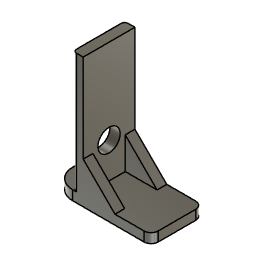
Improved Part (Autodesk Fusion 360 design; units mm, degrees)
Autodesk Fusion 360 part; units mm, degrees
sketch "Skizze1" plane through (0, 0, 0) normal (0, 0, 1) x (1, 0, 0)
  line L0 (-75, 50) -> (-47.27, 50)
  line L1 (-47.27, 50) -> (-47.27, 35.3603)
  line L2 (-47.27, 35.3603) -> (-75, 35.3603)
  line L3 (-75, 35.3603) -> (-75, 50)
  line L4 (-69.4, 50) -> (-69.4, 35.3603)
  line L5 (-66.5, 50) -> (-66.5, 35.3603)
  dimension "d1" = 27.73
  dimension "d2" = 5.6
  dimension "d3" = 2.9
  constraint horizontal L0
  constraint vertical L1
  constraint horizontal L2
  constraint vertical L3
  constraint coincident L0 L4.start
  constraint coincident L2 L4.end
  constraint perpendicular L2 L4
  constraint coincident L0 L5.start
  constraint coincident L2 L5.end
  constraint perpendicular L2 L5
  measures "d1" distance of L0.start L0.end
  measures "d2" distance of L3 L4
  measures "d3" distance of L4 L5
extrude "Extrusion1" add sketch "Skizze1" along normal blind 2.7 contours L0 L2 L3 L4 | L0 L1 L2 L5 makes body 1 at (-73.1333, 45.1201, 0) makes body 2 at (-60.09, 45.1201, 0)
extrude "Extrusion2" add sketch "Skizze1" along normal blind 36.7 contours L0 L2 L4 L5 bodies 1 2
sketch "Skizze2" plane through (-69.4, 0, 0) normal (-1, 0, 0) x (0, -1, 0)
  line L0 (-50, 2.7) -> (-35.3603, 2.7)
  line L1 (-35.3603, 2.7) -> (-35.3603, 36.7)
  line L2 (-35.3603, 36.7) -> (-50, 36.7)
  line L3 (-50, 36.7) -> (-50, 2.7)
  line L4 (-42.6802, 2.7) -> (-42.6802, 36.7) construction
  line L5 (-50, 12.7) -> (-35.3603, 12.7) construction
  line L6 (-50, 2.7) -> (-35.3603, 2.7) construction
  circle A0 centre (-42.6802, 12.7) radius 3.15
  dimension "d8" = 10
  dimension "d9" = 6.3
  constraint midpoint L0 L4.start
  constraint midpoint L2 L4.end
  constraint coincident L3 L5.start
  constraint coincident L1 L5.end
  constraint perpendicular L1 L5
  constraint midpoint L5 A0.centre
  measures "d8" distance of L5 L6
  measures "d9" diameter of A0
extrude "Extrusion3" cut sketch "Skizze2" against normal blind 3 contours A0 bodies 1
fillet "Abrundung1" radius 5.5 2 edges at (-75, 50, 1.35) (-75, 35.3603, 1.35) on bodies 1
sketch "Skizze3" plane through (0, 0, 2.7) normal (0, 0, 1) x (-1, 0, 0)
  line L0 (47.27, -50) -> (66.5, -50)
  line L1 (66.5, -50) -> (66.5, -35.3603)
  line L2 (66.5, -35.3603) -> (47.27, -35.3603)
  line L3 (47.27, -35.3603) -> (47.27, -50)
  line L4 (66.5, -38.1003) -> (47.27, -38.1003)
  line L5 (47.27, -47.26) -> (66.5, -47.26)
  line L6 (57.5, -38.1003) -> (57.5, -35.3603)
  line L7 (57.5, -47.26) -> (57.5, -50)
  dimension "d14" = 2.74
  dimension "d15" = 2.74
  dimension "d16" = 9
  dimension "d17" = 9
  constraint coincident L1 L4.start
  constraint coincident L3 L4.end
  constraint perpendicular L3 L4
  constraint coincident L3 L5.start
  constraint coincident L1 L5.end
  constraint perpendicular L1 L5
  constraint coincident L4 L6.start
  constraint coincident L2 L6.end
  constraint perpendicular L2 L6
  constraint coincident L5 L7.start
  constraint coincident L0 L7.end
  constraint perpendicular L0 L7
  measures "d14" distance of L2 L4
  measures "d15" distance of L0 L5
  measures "d16" distance of L1 L7
  measures "d17" distance of L1 L6
extrude "Extrusion4" add sketch "Skizze3" along normal blind 9 contours L0 L1 L5 L7 | L1 L2 L4 L6 bodies 1
chamfer "Fase2" distance 9 angle 45 2 edges at (-57.5, 36.7303, 11.7) (-57.5, 48.63, 11.7) on bodies 1
fillet "Abrundung2" radius 1 2 edges at (-69.4, 50, 19.7) (-69.4, 35.3603, 19.7) on bodies 1
fillet "Abrundung3" radius 2 2 edges at (-47.27, 50, 1.35) (-47.27, 35.3603, 1.35) on bodies 1
equation "d1 = 20 mm + 7.73 mm"
equation "d6 = 34 mm + 2.7 mm"
equation "d18 = 15 mm - 2.7 mm - 3.3 mm"
